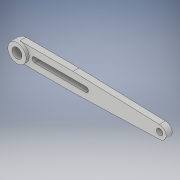
# Autodesk Inventor part: lever
Saved by Autodesk Inventor 2017.1 (Build 211199000, 199)
## iProperties
Created: 2017-05-25
Part Number: lever
Material: Generic
Document SubType Name: Modeling
Designer: 196918
Density: 1 g/cm^3
Appearance: Default
Author: 196918
Autodesk Inventor part; units mm, degrees
ref_plane "YZ Plane" through (0, 0, 0) normal (1, 0, 0) x (0, 1, 0)
ref_plane "XZ Plane" through (0, 0, 0) normal (0, 1, 0) x (-1, 0, 0)
sketch "Sketch1" plane through (0, 0, 0) normal (0, 0, 1) x (1, 0, 0)
  circle A0 centre (0, 0) radius 11.938
  line L0 (0, -11.938) -> (69.088, -11.938)
  line L1 (0, 11.938) -> (69.088, 11.938)
  line L2 (69.088, 11.938) -> (182.0608, 8.3422)
  line L3 (69.088, -11.938) -> (182.0608, -8.3422)
  arc A1 (181.2593, -8.3677) -> (181.2593, 8.3677) centre (181.7953, 0) ccw
  dimension "d0" = 23.876
  constraints: 8 end point, 4 point on circle, 2 centre point, 2 horizontal, 2 point on line, 1 coincident
  measures "d0" diameter of A0
extrude "Extrusion1" add sketch "Sketch1" along normal blind 11.684 contours A0
extrude "Extrusion2" add sketch "Sketch1" along normal blind 7.874 contours A0 L1 L2 A1 L3 L0
sketch "Sketch2" plane through (0, 0, 7.874) normal (0, 0, 1) x (1, 0, 0)
  line L0 (181.2593, 8.3677) -> (69.088, 11.938) projected
  arc A0 (181.2593, -8.3677) -> (181.2593, 8.3677) centre (181.7953, 0) ccw projected
  line L1 (69.088, -11.938) -> (181.2593, -8.3677) projected
  line L2 (69.088, 11.938) -> (0, 11.938) projected
  line L3 (0, -11.938) -> (69.088, -11.938) projected
  line L4 (69.088, -11.938) -> (181.2593, -8.3677) projected
  arc A1 (181.2593, -8.3677) -> (181.2593, 8.3677) centre (181.7953, 0) ccw projected
  line L5 (181.2593, 8.3677) -> (69.088, 11.938) projected
  line L6 (69.088, 11.938) -> (0, 11.938) projected
  arc A2 (0, -11.938) -> (0, 11.938) centre (0, 0) ccw projected
  circle A3 centre (181.7953, 0) radius 4.064
  line L7 (0, 0) -> (15.748, 0) construction
  line L8 (15.748, 0) -> (19.05, 0)
  arc A4 (19.05, 3.302) -> (19.05, -3.302) centre (19.05, 0) ccw
  line L9 (19.05, 3.302) -> (85.852, 3.302)
  arc A5 (85.852, -3.302) -> (85.852, 3.302) centre (85.852, 0) ccw
  line L10 (85.852, -3.302) -> (19.05, -3.302)
  dimension "d7" = 8.128
  dimension "d8" = 15.748
  dimension "d10" = 3.302
  dimension "d11" = 66.802
  constraints: 8 end point, 5 point on circle, 3 centre point, 3 horizontal, 3 tangent, 2 coincident
  measures "d7" diameter of A3
  measures "d8" distance of L7.start L7.end
  measures "d10" distance of L7.end L8.end
  measures "d11" distance of L9.start L9.end
extrude "Extrusion3" cut sketch "Sketch2" against normal up to next contours A3 | L9 A5 L10 A4
sketch "Sketch3" plane through (0, 0, 11.684) normal (0, 0, 1) x (1, 0, 0)
  circle A0 centre (0, 0) radius 6.477
  dimension "d14" = 12.954
  constraints: 1 centre point, 1 coincident
  measures "d14" diameter of A0
extrude "Extrusion4" cut sketch "Sketch3" against normal up to next
ref_plane "Work Plane1" through (0, 0, 3.937) normal (0, 0, 1) x (1, 0, 0)
body "Solid1"
